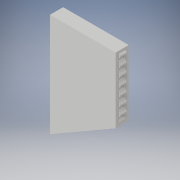
# Autodesk Inventor part: top right door
Saved by Autodesk Inventor 2017 (Build 210142000, 142)
## iProperties
Created: 2018-03-10
Part Number: top right door
Material: Generic
Document SubType Name: Modeling
Designer: Braxton
Density: 1 g/cm^3
Appearance: Default
Author: Braxton
Autodesk Inventor part; units mm, degrees
ref_plane "YZ Plane" through (0, 0, 0) normal (1, 0, 0) x (0, 1, 0)
ref_plane "XZ Plane" through (0, 0, 0) normal (0, 1, 0) x (-1, 0, 0)
ref_plane "XY Plane" through (0, 0, 0) normal (0, 0, 1) x (1, 0, 0)
sketch "Sketch1" plane through (0, 0, 0) normal (0, 0, 1) x (1, 0, 0)
  line L0 (1270, 1270) -> (0, 536.7652)
  line L1 (0, 536.7652) -> (0, 2540)
  line L2 (0, 2540) -> (1270, 2540)
  line L3 (1270, 1270) -> (1270, 2540)
  dimension "d446" = 2003.2348
  constraints: 8 end point, 1 perpendicular
  measures "d446" distance of L0.end L1.end
extrude "door" add sketch "Sketch1" along normal mid plane 254
sketch "Sketch3" plane through (0, 0, 0) normal (0, 0, 1) x (1, 0, 0)
  line L0 (33.8905, 585.6612) -> (71.1839, 577.8632)
  line L1 (35.592, 557.3142) -> (22.892, 579.3112) construction
  line L2 (11.8934, 572.9612) -> (33.8905, 585.6612)
  line L3 (11.8934, 572.9612) -> (0, 536.7652)
  line L4 (0, 536.7652) -> (71.1839, 577.8632)
  line L5 (71.1839, 577.8632) -> (108.4774, 570.0652)
  line L6 (108.4774, 570.0652) -> (130.4744, 582.7652)
  line L7 (130.4744, 582.7652) -> (142.3679, 618.9613)
  line L8 (1270, 1270) -> (0, 536.7652) projected
  line L9 (71.1839, 577.8632) -> (142.3679, 618.9613)
  line L10 (106.7759, 598.4123) -> (119.4759, 576.4152) construction
  line L11 (154.2613, 655.1574) -> (142.3679, 618.9613)
  line L12 (154.2613, 655.1574) -> (176.2584, 667.8574)
  line L13 (177.9598, 639.5103) -> (165.2598, 661.5074) construction
  line L14 (176.2584, 667.8574) -> (213.5518, 660.0593)
  line L15 (142.3679, 618.9613) -> (213.5518, 660.0593)
  line L16 (213.5518, 660.0593) -> (250.8452, 652.2613)
  line L17 (250.8452, 652.2613) -> (272.8423, 664.9613)
  line L18 (272.8423, 664.9613) -> (284.7357, 701.1574)
  line L19 (213.5518, 660.0593) -> (284.7357, 701.1574)
  line L20 (249.1438, 680.6084) -> (261.8438, 658.6113) construction
  line L21 (296.6292, 737.3535) -> (284.7357, 701.1574)
  line L22 (296.6292, 737.3535) -> (318.6262, 750.0535)
  line L23 (320.3277, 721.7064) -> (307.6277, 743.7035) construction
  line L24 (318.6262, 750.0535) -> (355.9197, 742.2555)
  line L25 (284.7357, 701.1574) -> (355.9197, 742.2555)
  line L26 (355.9197, 742.2555) -> (393.2131, 734.4575)
  line L27 (393.2131, 734.4575) -> (415.2102, 747.1575)
  line L28 (415.2102, 747.1575) -> (427.1036, 783.3535)
  line L29 (355.9197, 742.2555) -> (427.1036, 783.3535)
  line L30 (391.5116, 762.8045) -> (404.2116, 740.8075) construction
  line L31 (438.997, 819.5496) -> (427.1036, 783.3535)
  line L32 (438.997, 819.5496) -> (460.9941, 832.2496)
  line L33 (462.6956, 803.9026) -> (449.9956, 825.8996) construction
  line L34 (460.9941, 832.2496) -> (498.2875, 824.4516)
  line L35 (427.1036, 783.3535) -> (498.2875, 824.4516)
  line L36 (498.2875, 824.4516) -> (535.581, 816.6536)
  line L37 (535.581, 816.6536) -> (557.578, 829.3536)
  line L38 (557.578, 829.3536) -> (569.4715, 865.5497)
  line L39 (498.2875, 824.4516) -> (569.4715, 865.5497)
  line L40 (533.8795, 845.0006) -> (546.5795, 823.0036) construction
  line L41 (581.3649, 901.7457) -> (569.4715, 865.5497)
  line L42 (581.3649, 901.7457) -> (603.362, 914.4457)
  line L43 (605.0634, 886.0987) -> (592.3634, 908.0957) construction
  line L44 (603.362, 914.4457) -> (640.6554, 906.6477)
  line L45 (569.4715, 865.5497) -> (640.6554, 906.6477)
  line L46 (640.6554, 906.6477) -> (677.9488, 898.8497)
  line L47 (677.9488, 898.8497) -> (699.9459, 911.5497)
  line L48 (699.9459, 911.5497) -> (711.8393, 947.7458)
  line L49 (640.6554, 906.6477) -> (711.8393, 947.7458)
  line L50 (676.2474, 927.1968) -> (688.9474, 905.1997) construction
  line L51 (723.7328, 983.9419) -> (711.8393, 947.7458)
  line L52 (723.7328, 983.9419) -> (745.7298, 996.6419)
  line L53 (747.4313, 968.2948) -> (734.7313, 990.2919) construction
  line L54 (745.7298, 996.6419) -> (783.0233, 988.8439)
  line L55 (711.8393, 947.7458) -> (783.0233, 988.8439)
  line L56 (783.0233, 988.8439) -> (820.3167, 981.0458)
  line L57 (820.3167, 981.0458) -> (842.3138, 993.7458)
  line L58 (842.3138, 993.7458) -> (854.2072, 1029.9419)
  line L59 (783.0233, 988.8439) -> (854.2072, 1029.9419)
  line L60 (818.6152, 1009.3929) -> (831.3152, 987.3958) construction
  line L61 (866.1006, 1066.138) -> (854.2072, 1029.9419)
  line L62 (866.1006, 1066.138) -> (888.0977, 1078.838)
  line L63 (889.7992, 1050.4909) -> (877.0992, 1072.488) construction
  line L64 (888.0977, 1078.838) -> (925.3911, 1071.04)
  line L65 (854.2072, 1029.9419) -> (925.3911, 1071.04)
  line L66 (925.3911, 1071.04) -> (962.6846, 1063.242)
  line L67 (962.6846, 1063.242) -> (984.6816, 1075.942)
  line L68 (984.6816, 1075.942) -> (996.5751, 1112.138)
  line L69 (925.3911, 1071.04) -> (996.5751, 1112.138)
  line L70 (960.9831, 1091.589) -> (973.6831, 1069.592) construction
  line L71 (1008.4685, 1148.3341) -> (996.5751, 1112.138)
  line L72 (1008.4685, 1148.3341) -> (1030.4656, 1161.0341)
  line L73 (1032.167, 1132.6871) -> (1019.467, 1154.6841) construction
  line L74 (1030.4656, 1161.0341) -> (1067.759, 1153.2361)
  line L75 (996.5751, 1112.138) -> (1067.759, 1153.2361)
  line L76 (1067.759, 1153.2361) -> (1105.0525, 1145.4381)
  line L77 (1105.0525, 1145.4381) -> (1127.0495, 1158.1381)
  line L78 (1127.0495, 1158.1381) -> (1138.9429, 1194.3342)
  line L79 (1067.759, 1153.2361) -> (1138.9429, 1194.3342)
  line L80 (1103.351, 1173.7851) -> (1116.051, 1151.7881) construction
  line L81 (1172.8334, 1243.2302) -> (1210.1269, 1235.4322)
  line L82 (1174.5349, 1214.8832) -> (1161.8349, 1236.8802) construction
  line L83 (1150.8364, 1230.5302) -> (1172.8334, 1243.2302)
  line L84 (1150.8364, 1230.5302) -> (1138.9429, 1194.3342)
  line L85 (1138.9429, 1194.3342) -> (1210.1269, 1235.4322)
  line L86 (1295.4, 2436.0832) -> (1270, 2407.6852)
  line L87 (1295.4, 2461.4832) -> (1295.4, 2436.0832)
  line L88 (1270, 2448.7832) -> (1295.4, 2448.7832) construction
  line L89 (1270, 2489.8813) -> (1270, 2407.6852)
  line L90 (1270, 2489.8813) -> (1295.4, 2461.4832)
  line L91 (1295.4, 2271.691) -> (1270, 2243.2929)
  line L92 (1295.4, 2297.091) -> (1295.4, 2271.691)
  line L93 (1270, 2284.391) -> (1295.4, 2284.391) construction
  line L94 (1270, 2325.4891) -> (1270, 2243.2929)
  line L95 (1270, 2325.4891) -> (1295.4, 2297.091)
  line L96 (1244.6, 2353.8871) -> (1270, 2325.4891)
  line L97 (1270, 2366.5871) -> (1244.6, 2366.5871) construction
  line L98 (1244.6, 2379.2871) -> (1244.6, 2353.8871)
  line L99 (1244.6, 2379.2871) -> (1270, 2407.6852)
  line L100 (1270, 2407.6852) -> (1270, 2325.4891)
  line L101 (1295.4, 2107.2987) -> (1270, 2078.9007)
  line L102 (1295.4, 2132.6987) -> (1295.4, 2107.2987)
  line L103 (1270, 2119.9987) -> (1295.4, 2119.9987) construction
  line L104 (1270, 2161.0968) -> (1270, 2078.9007)
  line L105 (1270, 2161.0968) -> (1295.4, 2132.6987)
  line L106 (1244.6, 2189.4949) -> (1270, 2161.0968)
  line L107 (1270, 2202.1949) -> (1244.6, 2202.1949) construction
  line L108 (1244.6, 2214.8949) -> (1244.6, 2189.4949)
  line L109 (1244.6, 2214.8949) -> (1270, 2243.2929)
  line L110 (1270, 2243.2929) -> (1270, 2161.0968)
  line L111 (1295.4, 1942.9065) -> (1270, 1914.5084)
  line L112 (1295.4, 1968.3065) -> (1295.4, 1942.9065)
  line L113 (1270, 1955.6065) -> (1295.4, 1955.6065) construction
  line L114 (1270, 1996.7045) -> (1270, 1914.5084)
  line L115 (1270, 1996.7045) -> (1295.4, 1968.3065)
  line L116 (1244.6, 2025.1026) -> (1270, 1996.7045)
  line L117 (1270, 2037.8026) -> (1244.6, 2037.8026) construction
  line L118 (1244.6, 2050.5026) -> (1244.6, 2025.1026)
  line L119 (1244.6, 2050.5026) -> (1270, 2078.9007)
  line L120 (1270, 2078.9007) -> (1270, 1996.7045)
  line L121 (1295.4, 1778.5142) -> (1270, 1750.1162)
  line L122 (1295.4, 1803.9142) -> (1295.4, 1778.5142)
  line L123 (1270, 1791.2142) -> (1295.4, 1791.2142) construction
  line L124 (1270, 1832.3123) -> (1270, 1750.1162)
  line L125 (1270, 1832.3123) -> (1295.4, 1803.9142)
  line L126 (1244.6, 1860.7104) -> (1270, 1832.3123)
  line L127 (1270, 1873.4104) -> (1244.6, 1873.4104) construction
  line L128 (1244.6, 1886.1104) -> (1244.6, 1860.7104)
  line L129 (1244.6, 1886.1104) -> (1270, 1914.5084)
  line L130 (1270, 1914.5084) -> (1270, 1832.3123)
  line L131 (1295.4, 1614.122) -> (1270, 1585.7239)
  line L132 (1295.4, 1639.522) -> (1295.4, 1614.122)
  line L133 (1270, 1626.822) -> (1295.4, 1626.822) construction
  line L134 (1270, 1667.92) -> (1270, 1585.7239)
  line L135 (1270, 1667.92) -> (1295.4, 1639.522)
  line L136 (1244.6, 1696.3181) -> (1270, 1667.92)
  line L137 (1270, 1709.0181) -> (1244.6, 1709.0181) construction
  line L138 (1244.6, 1721.7181) -> (1244.6, 1696.3181)
  line L139 (1244.6, 1721.7181) -> (1270, 1750.1162)
  line L140 (1270, 1750.1162) -> (1270, 1667.92)
  line L141 (1295.4, 1449.7297) -> (1270, 1421.3317)
  line L142 (1295.4, 1475.1297) -> (1295.4, 1449.7297)
  line L143 (1270, 1462.4297) -> (1295.4, 1462.4297) construction
  line L144 (1270, 1503.5278) -> (1270, 1421.3317)
  line L145 (1270, 1503.5278) -> (1295.4, 1475.1297)
  line L146 (1244.6, 1531.9258) -> (1270, 1503.5278)
  line L147 (1270, 1544.6258) -> (1244.6, 1544.6258) construction
  line L148 (1244.6, 1557.3258) -> (1244.6, 1531.9258)
  line L149 (1244.6, 1557.3258) -> (1270, 1585.7239)
  line L150 (1270, 1585.7239) -> (1270, 1503.5278)
  line L151 (1244.6, 1392.9336) -> (1270, 1421.3317)
  line L152 (1270, 1380.2336) -> (1244.6, 1380.2336) construction
  line L153 (1244.6, 1392.9336) -> (1244.6, 1367.5336)
  line L154 (1270, 1421.3317) -> (1270, 1339.1355)
  line L155 (1244.6, 1367.5336) -> (1270, 1339.1355)
  line L156 (0, 536.7652) -> (0, 2540) projected
  dimension "d282" = 25.4
  dimension "d283" = 25.4
  dimension "d284" = 38.1
  dimension "d285" = 38.1
  dimension "d350" = 38.1
  dimension "d351" = 25.4
  dimension "d352" = 38.1
  dimension "d353" = 138.19
  dimension "d356" = 138.19
  dimension "d358" = 25.4
  dimension "d359" = 25.4
  dimension "d360" = 25.4
  dimension "d361" = 38.1
  dimension "d362" = 38.1
  dimension "d363" = 38.1
  dimension "d364" = 25.4
  dimension "d365" = 38.1
  dimension "d366" = 138.19
  dimension "d367" = 138.19
  dimension "d368" = 25.4
  dimension "d369" = 25.4
  dimension "d370" = 25.4
  dimension "d371" = 38.1
  dimension "d372" = 38.1
  dimension "d373" = 38.1
  dimension "d374" = 25.4
  dimension "d375" = 38.1
  dimension "d376" = 138.19
  dimension "d377" = 138.19
  dimension "d378" = 25.4
  dimension "d379" = 25.4
  dimension "d380" = 25.4
  dimension "d381" = 38.1
  dimension "d382" = 38.1
  dimension "d383" = 38.1
  dimension "d384" = 25.4
  dimension "d385" = 38.1
  dimension "d386" = 138.19
  dimension "d387" = 138.19
  dimension "d388" = 25.4
  dimension "d389" = 25.4
  dimension "d390" = 25.4
  dimension "d391" = 38.1
  dimension "d392" = 38.1
  dimension "d393" = 38.1
  dimension "d394" = 25.4
  dimension "d395" = 38.1
  dimension "d396" = 138.19
  dimension "d397" = 138.19
  dimension "d398" = 25.4
  dimension "d399" = 25.4
  dimension "d400" = 25.4
  dimension "d401" = 38.1
  dimension "d402" = 38.1
  dimension "d403" = 38.1
  dimension "d404" = 25.4
  dimension "d405" = 38.1
  dimension "d406" = 138.19
  dimension "d407" = 138.19
  dimension "d408" = 25.4
  dimension "d409" = 25.4
  dimension "d410" = 25.4
  dimension "d411" = 38.1
  dimension "d412" = 38.1
  constraints: 310 end point, 25 midpoint, 18 perpendicular, 16 collinear
  measures "d282" distance of L1.start L1.end
  measures "d283" distance of L3.start L2.end
  measures "d284" distance of L3.end L3.start
  measures "d285" distance of L2.end L0.end
  measures "d350" distance of L0.end L5.end
  measures "d351" distance of L5.end L6.end
  measures "d352" distance of L7.end L6.end
  measures "d353" angle of L2 L3
  measures "d356" angle of L6 L5
  measures "d358" distance of L10.start L10.end
  measures "d359" distance of L13.start L13.end
  measures "d360" distance of L12.start L14.start
  measures "d361" distance of L7.end L12.start
  measures "d362" distance of L14.start L19.start
  measures "d363" distance of L19.start L17.start
  measures "d364" distance of L17.start L18.start
  measures "d365" distance of L18.end L18.start
  measures "d366" angle of L12 L11
  measures "d367" angle of L17 L16
  measures "d368" distance of L20.start L20.end
  measures "d369" distance of L23.start L23.end
  measures "d370" distance of L22.start L24.start
  measures "d371" distance of L18.end L22.start
  measures "d372" distance of L24.start L29.start
  measures "d373" distance of L29.start L27.start
  measures "d374" distance of L27.start L28.start
  measures "d375" distance of L28.end L28.start
  measures "d376" angle of L22 L21
  measures "d377" angle of L27 L26
  measures "d378" distance of L30.start L30.end
  measures "d379" distance of L33.start L33.end
  measures "d380" distance of L32.start L34.start
  measures "d381" distance of L28.end L32.start
  measures "d382" distance of L34.start L39.start
  measures "d383" distance of L39.start L37.start
  measures "d384" distance of L37.start L38.start
  measures "d385" distance of L38.end L38.start
  measures "d386" angle of L32 L31
  measures "d387" angle of L37 L36
  measures "d388" distance of L40.start L40.end
  measures "d389" distance of L43.start L43.end
  measures "d390" distance of L42.start L44.start
  measures "d391" distance of L38.end L42.start
  measures "d392" distance of L44.start L49.start
  measures "d393" distance of L49.start L47.start
  measures "d394" distance of L47.start L48.start
  measures "d395" distance of L48.end L48.start
  measures "d396" angle of L42 L41
  measures "d397" angle of L47 L46
  measures "d398" distance of L50.start L50.end
  measures "d399" distance of L53.start L53.end
  measures "d400" distance of L52.start L54.start
  measures "d401" distance of L48.end L52.start
  measures "d402" distance of L54.start L59.start
  measures "d403" distance of L59.start L57.start
  measures "d404" distance of L57.start L58.start
  measures "d405" distance of L58.end L58.start
  measures "d406" angle of L52 L51
  measures "d407" angle of L57 L56
  measures "d408" distance of L60.start L60.end
  measures "d409" distance of L63.start L63.end
  measures "d410" distance of L62.start L64.start
  measures "d411" distance of L58.end L62.start
  measures "d412" distance of L64.start L69.start
extrude "connection give" cut sketch "Sketch3" along normal mid plane 127 contours L84 L83 L81 L8 | L71 L72 L74 L8 | L61 L62 L64 L8 | L51 L52 L54 L8 | L41 L42 L44 L8 | L31 L32 L34 L8 | L21 L22 L24 L8 | L11 L12 L14 L8 | L0 L4 L3 L2 | L154 L155 L153 L151 | L150 L146 L148 L149 | L140 L136 L138 L139 | L130 L126 L128 L129 | L120 L116 L118 L119 | L110 L106 L108 L109 | L100 L96 L98 L99
extrude "connection receive" add sketch "Sketch3" along normal mid plane 127 contours L8 L78 L77 L76 | L8 L68 L67 L66 | L8 L58 L57 L56 | L8 L48 L47 L46 | L8 L38 L37 L36 | L8 L28 L27 L26 | L8 L18 L17 L16 | L8 L7 L6 L5 | L145 L142 L141 L144 | L135 L132 L131 L134 | L125 L122 L121 L124 | L115 L112 L111 L114 | L105 L102 L101 L104 | L95 L92 L91 L94 | L86 L89 L90 L87
body "Solid1"
